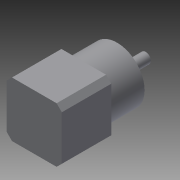
# Autodesk Inventor part: ExtruderMotor
Saved by Autodesk Inventor 2014 SP1 (Build 180222100, 222)
## iProperties
Created: 2014-01-05
Part Number: ExtruderMotor
Material: Generic
Document SubType Name: Modeling
Designer: Jack
Density: 1 g/cm^3
Appearance: Default
Author: Jack
Autodesk Inventor part; units mm, degrees
ref_plane "YZ Plane" through (0, 0, 0) normal (1, 0, 0) x (0, 1, 0)
ref_plane "XZ Plane" through (0, 0, 0) normal (0, 1, 0) x (-1, 0, 0)
ref_plane "XY Plane" through (0, 0, 0) normal (0, 0, 1) x (1, 0, 0)
sketch "Sketch1" plane through (0, 0, 0) normal (0, 1, 0) x (-1, 0, 0)
  line L0 (4, 0) -> (38.3, 0)
  line L1 (42.3, 4) -> (42.3, 38.3)
  line L2 (38.3, 42.3) -> (4, 42.3)
  line L3 (0, 38.3) -> (0, 4)
  line L4 (0, 38.3) -> (4, 42.3)
  line L5 (42.3, 38.3) -> (38.3, 42.3)
  line L6 (38.3, 0) -> (42.3, 4)
  line L7 (4, 0) -> (0, 4)
  point P0 (0, 0)
  point P1 (42.3, 0)
  point P2 (42.3, 42.3)
  point P3 (0, 42.3)
  dimension "d0" = 42.3
  dimension "d1" = 42.3
  dimension "d2" = 4
  dimension "d3" = 4
  dimension "d4" = 4
  dimension "d5" = 4
  dimension "d6" = 4
  dimension "d7" = 4
  dimension "d8" = 4
  dimension "d9" = 4
  constraints: 16 end point, 8 point on line, 3 perpendicular, 1 horizontal
  measures "d0" distance of point (0, 0) point (42.3, 0)
  measures "d1" distance of point (42.3, 0) point (42.3, 42.3)
  measures "d2" distance of L3.start point (0, 42.3)
  measures "d3" distance of L2.end point (0, 42.3)
  measures "d4" distance of L1.end point (42.3, 42.3)
  measures "d5" distance of L2.start point (42.3, 42.3)
  measures "d6" distance of L0.end point (42.3, 0)
  measures "d7" distance of L1.start point (42.3, 0)
  measures "d8" distance of L0.start point (0, 0)
  measures "d9" distance of L3.end point (0, 0)
extrude "Extrusion1" add sketch "Sketch1" along normal blind 38
sketch "Sketch2" plane through (0, 38, 0) normal (0, 1, 0) x (1, 0, 0)
  line L0 (-4, 0) -> (-38.3, 0) projected
  line L1 (-42.3, -4) -> (-42.3, -38.3) projected
  circle A0 centre (-36.65, -5.65) radius 1.5
  circle A1 centre (-5.65, -5.65) radius 1.5
  circle A2 centre (-5.65, -36.65) radius 1.5
  circle A3 centre (-36.65, -36.65) radius 1.5
  point P0 (0, 0)
  dimension "d12" = 3
  dimension "d13" = 3
  dimension "d14" = 3
  dimension "d15" = 3
  dimension "d17" = 31
  dimension "d18" = 5.65
  dimension "d19" = 5.65
  dimension "d20" = 31
  constraints: 4 centre point, 2 horizontal alignment, 2 vertical alignment
  measures "d12" diameter of A0
  measures "d13" diameter of A1
  measures "d14" diameter of A2
  measures "d15" diameter of A3
  measures "d17" distance of A2.centre A3.centre
  measures "d18" distance from line of L0 A0.centre
  measures "d19" distance from line of L1 A3.centre
  measures "d20" distance of A1.centre A2.centre
extrude "Extrusion2" cut sketch "Sketch2" against normal blind 4
thread "Thread1" size "M3x0.5" class "6H" standard "ANSI Metric M Profile" full length
thread "Thread2" size "M3x0.5" class "6H" standard "ANSI Metric M Profile" full length
thread "Thread3" size "M3x0.5" class "6H" standard "ANSI Metric M Profile" full length
thread "Thread4" size "M3x0.5" class "6H" standard "ANSI Metric M Profile" full length
sketch "Sketch3" plane through (0, 38, 0) normal (0, 1, 0) x (1, 0, 0)
  line L0 (0, -38.3) -> (0, -4) projected
  line L1 (-38.3, -42.3) -> (-4, -42.3) projected
  circle A0 centre (-21.15, -21.15) radius 21.15
  point P0 (0, 0)
  dimension "d31" = 21.15
  dimension "d32" = 21.15
  dimension "d33" = 42.3
  constraints: 1 centre point
  measures "d31" distance from line of L1 A0.centre
  measures "d32" distance from line of L0 A0.centre
  measures "d33" diameter of A0
extrude "Extrusion3" add sketch "Sketch3" along normal blind 25.6
sketch "Sketch4" plane through (-21.15, 63.6, 21.15) normal (0, 1, 0) x (1, 0, 0)
  circle A0 centre (0, 0) radius 21.15 projected
  circle A1 centre (0, 0) radius 17.5 construction
  line L0 (0, 0) -> (12.3744, 12.3744) construction
  line L1 (0, 0) -> (12.3744, -12.3744) construction
  line L2 (0, 0) -> (-12.3744, -12.3744) construction
  line L3 (0, 0) -> (-12.3744, 12.3744) construction
  line L4 (-17.5, 0) -> (17.5, 0) construction
  circle A2 centre (12.3744, 12.3744) radius 2
  circle A3 centre (12.3744, -12.3744) radius 2
  circle A4 centre (-12.3744, -12.3744) radius 2
  circle A5 centre (-12.3744, 12.3744) radius 2
  point P0 (21.15, 21.15)
  dimension "d36" = 35
  dimension "d37" = 45
  dimension "d38" = 45
  dimension "d39" = 4
  dimension "d40" = 4
  dimension "d41" = 4
  dimension "d42" = 4
  constraints: 10 end point, 6 point on circle, 5 centre point, 5 coincident, 2 perpendicular, 1 horizontal, 1 midpoint
  measures "d36" diameter of A1
  measures "d37" angle of L0 L4
  measures "d38" angle of L4 L3
  measures "d39" diameter of A2
  measures "d40" diameter of A3
  measures "d41" diameter of A4
  measures "d42" diameter of A5
extrude "Extrusion4" cut sketch "Sketch4" against normal blind 6 contours A2 | A3 | A4 | A5
thread "Thread5" size "M4x0.7" class "6H" standard "ANSI Metric M Profile" full length
thread "Thread6" size "M4x0.7" class "6H" standard "ANSI Metric M Profile" full length
thread "Thread7" size "M4x0.7" class "6H" standard "ANSI Metric M Profile" full length
thread "Thread8" size "M4x0.7" class "6H" standard "ANSI Metric M Profile" full length
sketch "Sketch5" plane through (-21.15, 63.6, 21.15) normal (0, 1, 0) x (1, 0, 0)
  circle A0 centre (0, 0) radius 21.15 projected
  line L0 (11.4, -5.1274) -> (11.4, 5.1274)
  line L1 (-11.4, 5.1274) -> (-11.4, -5.1274)
  arc A1 (11.4, 5.1274) -> (-11.4, 5.1274) centre (0, 0) ccw
  arc A2 (-11.4, -5.1274) -> (11.4, -5.1274) centre (0, 0) ccw
  point P0 (21.15, 21.15)
  dimension "d54" = 11.4
  dimension "d55" = 11.4
  dimension "d56" = 12.5
  dimension "d57" = 12.5
  constraints: 4 end point, 4 point on circle, 2 centre point, 1 coincident, 1 parallel, 1 vertical
  measures "d54" distance from line of A1.centre L1
  measures "d55" distance from line of A0.centre L0
  measures "d56" radius of A1
  measures "d57" radius of A2
extrude "Extrusion5" add sketch "Sketch5" along normal blind 2 contours A2 L1 A1 L0
sketch "Sketch6" plane through (-21.15, 65.6, 21.15) normal (0, 1, 0) x (1, 0, 0)
  arc A0 (-11.4, -5.1274) -> (11.4, -5.1274) centre (0, 0) ccw projected
  circle A1 centre (0, 0) radius 4
  point P0 (21.15, 21.15)
  dimension "d60" = 8
  constraints: 1 centre point, 1 coincident
  measures "d60" diameter of A1
extrude "Extrusion6" add sketch "Sketch6" along normal blind 20
sketch "Sketch7" plane through (-21.15, 85.6, 21.15) normal (0, 1, 0) x (1, 0, 0)
  circle A0 centre (0, 0) radius 4 projected
  line L0 (-2.6458, 3) -> (2.6458, 3)
  point P0 (21.15, 21.15)
  dimension "d63" = 7
  constraints: 2 end point, 2 point on circle, 1 horizontal
extrude "Extrusion7" cut sketch "Sketch7" against normal blind 15 contours L0 A0 picked at (-0.6179, 3.1815)
equation "\"d3\" = d2"
equation "\"d4\" = d2"
equation "\"d5\" = d4"
equation "\"d6\" = d2"
equation "\"d7\" = d6"
equation "\"d8\" = d2"
equation "\"d9\" = d8"
body "Solid1"
